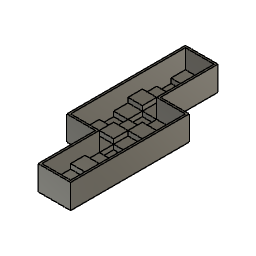
Stepfields v1 (Autodesk Fusion 360 design; units mm, degrees)
Autodesk Fusion 360 part; units mm, degrees
sketch "Sketch1" plane through (0, 0, 0) normal (0, 0, 1) x (1, 0, 0)
  line L0 (0, 0) -> (300, 0)
  line L1 (300, 0) -> (300, 1200)
  line L2 (300, 1200) -> (0, 1200)
  line L3 (0, 600) -> (-300, 600)
  line L4 (-300, 600) -> (-300, 1800)
  line L5 (-300, 1800) -> (0, 1800)
  line L6 (0, 1800) -> (0, 1200)
  line L7 (0, 0) -> (0, 600)
  line L8 (20, 1820) -> (20, 1220)
  line L9 (320, 1220) -> (20, 1220)
  line L10 (320, -20) -> (320, 1220)
  line L11 (-20, -20) -> (320, -20)
  line L12 (-20, -20) -> (-20, 580)
  line L13 (-20, 580) -> (-320, 580)
  line L14 (-320, 580) -> (-320, 1820)
  line L15 (-320, 1820) -> (20, 1820)
  dimension "d1" = 300
  dimension "d2" = 1200
  dimension "d3" = 300
  dimension "d4" = 1200
  dimension "d5" = -20
  constraint horizontal L0
  constraint vertical L1
  constraint horizontal L2
  constraint coincident L0.start L7.start
  constraint perpendicular L3 L4
  constraint perpendicular L4 L5
  constraint perpendicular L2 L6
  constraint perpendicular L3 L7
  measures "d1" distance of L0.start L0.end
  measures "d2" distance of L0.end L1.end
  measures "d3" distance of L3.start L3.end
  measures "d4" distance of L3.end L4.end
extrude "Extrude1" add sketch "Sketch1" along normal blind 400 makes body 1
extrude "Extrude2" add sketch "Sketch1" against normal blind 5 separate body contours L0 L1 L2 L3 L4 L5 L6 L7 makes body 2
extrude "Extrude3" add sketch "Sketch1" against normal blind 5 bodies 1 2
extrude "Extrude4" cut 1 faces at (-313.3333, 1400, 400) along direction (0, 0, -1) blind 100 on bodies 1 bodies 1
extrude "Extrude5" cut 1 faces at (-313.3333, 1400, 300) along direction (0, 0, -1) blind 50 on bodies 1 bodies 1
sketch "Sketch2" plane through (0, 0, 0) normal (0, 0, 1) x (1, 0, 0)
  line L0 (0, 0) -> (150, 0)
  line L1 (150, 0) -> (150, 150)
  line L2 (150, 150) -> (0, 150)
  line L3 (0, 150) -> (0, 0)
  line L4 (150, 150) -> (300, 150)
  line L5 (300, 150) -> (300, 0)
  line L6 (300, 0) -> (150, 0)
  line L7 (0, 300) -> (150, 300)
  line L8 (0, 150) -> (0, 300)
  line L9 (150, 300) -> (150, 150)
  line L10 (300, 300) -> (150, 300)
  line L11 (300, 150) -> (300, 300)
  line L12 (150, 600) -> (150, 450)
  line L13 (150, 450) -> (0, 450)
  line L14 (150, 450) -> (300, 450)
  line L15 (150, 300) -> (150, 450)
  line L16 (0, 600) -> (150, 600)
  line L17 (0, 450) -> (0, 600)
  line L18 (300, 600) -> (150, 600)
  line L19 (0, 450) -> (0, 300)
  line L20 (300, 450) -> (300, 300)
  line L21 (300, 450) -> (300, 600)
  line L22 (0, 1200) -> (150, 1200)
  line L23 (0, 1050) -> (0, 900)
  line L24 (300, 1200) -> (150, 1200)
  line L25 (150, 900) -> (150, 1050)
  line L26 (150, 750) -> (0, 750)
  line L27 (0, 900) -> (150, 900)
  line L28 (300, 1050) -> (300, 1200)
  line L29 (150, 900) -> (150, 750)
  line L30 (0, 750) -> (0, 900)
  line L31 (300, 750) -> (300, 600)
  line L32 (150, 1050) -> (0, 1050)
  line L33 (150, 750) -> (300, 750)
  line L34 (300, 1050) -> (300, 900)
  line L35 (150, 1050) -> (300, 1050)
  line L36 (150, 600) -> (150, 750)
  line L37 (0, 1050) -> (0, 1200)
  line L38 (300, 900) -> (150, 900)
  line L39 (300, 750) -> (300, 900)
  line L40 (150, 1200) -> (150, 1050)
  line L41 (0, 750) -> (0, 600)
  line L42 (-150, 900) -> (-150, 750)
  line L43 (0, 900) -> (-150, 900)
  line L44 (-150, 750) -> (0, 750)
  line L45 (-150, 600) -> (-150, 750)
  line L46 (-150, 900) -> (-150, 1050)
  line L47 (-300, 1200) -> (-150, 1200)
  line L48 (-300, 750) -> (-300, 900)
  line L49 (-300, 1050) -> (-300, 1200)
  line L50 (-150, 1050) -> (0, 1050)
  line L51 (-150, 1050) -> (-300, 1050)
  line L52 (-300, 1050) -> (-300, 900)
  line L53 (0, 1200) -> (-150, 1200)
  line L54 (-150, 1200) -> (-150, 1050)
  line L55 (0, 600) -> (-150, 600)
  line L56 (-300, 900) -> (-150, 900)
  line L57 (-300, 750) -> (-300, 600)
  line L58 (-300, 600) -> (-150, 600)
  line L59 (-300, 1650) -> (-300, 1800)
  line L60 (-300, 1650) -> (-300, 1500)
  line L61 (0, 1650) -> (0, 1500)
  line L62 (-150, 1650) -> (0, 1650)
  line L63 (-150, 1500) -> (-150, 1650)
  line L64 (-300, 1350) -> (-300, 1500)
  line L65 (-150, 1500) -> (-150, 1350)
  line L66 (0, 1350) -> (0, 1500)
  line L67 (-150, 1350) -> (-300, 1350)
  line L68 (0, 1350) -> (0, 1200)
  line L69 (-300, 1350) -> (-300, 1200)
  line L70 (-150, 1800) -> (-150, 1650)
  line L71 (-300, 1500) -> (-150, 1500)
  line L72 (0, 1500) -> (-150, 1500)
  line L73 (-150, 1350) -> (0, 1350)
  line L74 (-300, 1800) -> (-150, 1800)
  line L75 (-150, 1200) -> (-150, 1350)
  line L76 (0, 1800) -> (-150, 1800)
  line L77 (0, 1650) -> (0, 1800)
  line L78 (-300, 750) -> (-150, 750)
  line L79 (-300, 1650) -> (-150, 1650)
  point P0 (0, 1200)
  point P1 (150, 600)
  point P2 (0, 900)
  point P3 (0, 600)
  point P4 (0, 750)
  point P5 (-150, 600)
  point P6 (-150, 750)
  point P7 (0, 1050)
  point P8 (0, 1350)
  point P9 (-150, 1200)
  point P10 (0, 1500)
  point P11 (-150, 1800)
  point P12 (-150, 1650)
  point P13 (0, 1200)
  point P14 (0, 1200)
  dimension "d16" = 150
  dimension "d17" = 150
  constraint horizontal L0
  constraint vertical L1
  constraint horizontal L2
  constraint vertical L3
  constraint coincident L0.start L3.end
  constraint symmetric L0.start L1 L5.end
  constraint symmetric L0.end L1 L6.end
  constraint symmetric L2.start L1 L4.start
  constraint symmetric L2.end L1 L4.end
  constraint symmetric L0.start L2 L7.start
  constraint symmetric L0.end L2 L7.end
  constraint symmetric L1.end L2 L4.start
  constraint symmetric L3.start L2 L8.start
  constraint symmetric L2 L4.end L5.start
  constraint symmetric L2 L5.end L10.start
  constraint symmetric L2 L0.end L7.end
  constraint symmetric L0.start L7 P3
  constraint symmetric L0.end L7 P1
  constraint symmetric L1.end L7 L12.end
  constraint symmetric L2.end L7 L13.end
  constraint symmetric L4.end L7 L14.end
  constraint symmetric L5.end L7 L18.start
  constraint symmetric L8.end L7 L19.end
  constraint symmetric L9.start L7 L10.end
  constraint symmetric L7 L2.end L13.end
  constraint symmetric L7 L1.end L12.end
  constraint symmetric L7 L10.start L11.end
  constraint symmetric L7 L4.end L14.end
  constraint symmetric L0.start L16 P14
  constraint symmetric L0.end L16 L22.end
  constraint symmetric L1.end L16 L25.end
  constraint symmetric L2.end L16 P7
  constraint symmetric L4.end L16 L28.start
  constraint symmetric L5.end L16 L24.start
  constraint symmetric L7.start L16 P2
  constraint symmetric L7.end L16 L25.start
  constraint symmetric L10.start L16 L34.end
  constraint symmetric P1 L16 L12.start
  constraint symmetric L12.end L16 L26.start
  constraint symmetric L13.end L16 P4
  constraint symmetric L14.end L16 L31.start
  constraint symmetric P3 L16 L17.end
  constraint symmetric L16 L18.start L21.end
  constraint symmetric L16 P1 L12.start
  constraint symmetric L16 L13.end P4
  constraint symmetric L16 L7.start P2
  constraint symmetric L16 L14.end L31.start
  constraint symmetric L16 L10.start L34.end
  constraint symmetric P1 L30 P5
  constraint symmetric P3 L30 L16.start
  constraint symmetric L18.start L30 L57.end
  constraint symmetric P14 L30 P13
  constraint symmetric P7 L30 L23.start
  constraint symmetric L25.end L30 L46.end
  constraint symmetric L22.end L30 P9
  constraint symmetric L34.end L30 L48.end
  constraint symmetric L25.start L30 L42.start
  constraint symmetric L28.start L30 L49.start
  constraint symmetric P4 L30 L26.end
  constraint symmetric L26.start L30 P6
  constraint symmetric P2 L30 L23.end
  constraint symmetric L31.start L30 L48.start
  constraint symmetric L24.start L30 L47.start
  constraint symmetric P14 L47 P13
  constraint symmetric P7 L47 P8
  constraint symmetric P4 L47 L61.start
  constraint symmetric P2 L47 P10
  constraint symmetric P3 L47 L76.start
  constraint symmetric P5 L47 P11
  constraint symmetric L49.start L47 L64.start
  constraint symmetric L46.end L47 L65.end
  constraint symmetric P6 L47 P12
  constraint symmetric L48.start L47 L59.start
  constraint symmetric P9 L47 L53.end
  constraint symmetric L48.end L47 L60.end
  constraint symmetric L42.start L47 L63.start
  constraint symmetric L49.end L47 L69.end
  constraint symmetric L47 P14 P13
  constraint symmetric L47 L57.end L59.end
  measures "d16" distance of L0.start L0.end
  measures "d17" distance of L0.end L1.end
extrude "Extrude6" add sketch "Sketch2" along normal blind 50 separate body contours L59 L70 L74 L79 makes body 3
extrude "Extrude7" add sketch "Sketch2" along normal blind 50 separate body contours L64 L65 L67 L71 makes body 4
extrude "Extrude8" add sketch "Sketch2" along normal blind 100 contours L47 L67 L69 L75 bodies 4
extrude "Extrude9" add sketch "Sketch2" along normal blind 50 contours L47 L49 L51 L54 bodies 4
extrude "Extrude10" add sketch "Sketch2" along normal blind 50 separate body contours L42 L48 L56 L78 makes body 5
extrude "Extrude11" add sketch "Sketch2" along normal blind 100 contours L45 L57 L58 L78 bodies 5
extrude "Extrude12" add sketch "Sketch2" along normal blind 50 separate body contours L61 L62 L63 L72 makes body 6
extrude "Extrude13" add sketch "Sketch2" along normal blind 100 contours L65 L66 L72 L73 bodies 6 4
extrude "Extrude14" add sketch "Sketch2" along normal blind 50 separate body contours L53 L68 L73 L75 makes body 7
extrude "Extrude15" add sketch "Sketch2" along normal blind 50 separate body contours L23 L43 L46 L50 makes body 8
extrude "Extrude16" add sketch "Sketch2" along normal blind 100 contours L30 L42 L43 L44 bodies 8 5
extrude "Extrude17" add sketch "Sketch2" along normal blind 50 separate body contours L41 L44 L45 L55 makes body 9
extrude "Extrude18" add sketch "Sketch2" along normal blind 50 separate body contours L22 L32 L37 L40 makes body 10
extrude "Extrude19" add sketch "Sketch2" along normal blind 100 contours L24 L28 L35 L40 bodies 10
extrude "Extrude20" add sketch "Sketch2" along normal blind 50 contours L25 L34 L35 L38 bodies 10
extrude "Extrude21" add sketch "Sketch2" along normal blind 50 separate body contours L18 L31 L33 L36 makes body 11
extrude "Extrude22" add sketch "Sketch2" along normal blind 100 contours L12 L14 L18 L21 bodies 11
extrude "Extrude23" add sketch "Sketch2" along normal blind 50 contours L10 L14 L15 L20 bodies 11
extrude "Extrude24" add sketch "Sketch2" along normal blind 50 separate body contours L1 L4 L5 L6 makes body 12
extrude "Extrude25" add sketch "Sketch2" along normal blind 100 separate body contours L23 L25 L27 L32 makes body 13
extrude "Extrude26" add sketch "Sketch2" along normal blind 50 contours L26 L27 L29 L30 bodies 13 8 9 10 11
extrude "Extrude27" add sketch "Sketch2" along normal blind 50 separate body contours L12 L13 L16 L17 makes body 14
extrude "Extrude28" add sketch "Sketch2" along normal blind 100 contours L7 L13 L15 L19 bodies 14 13
extrude "Extrude29" add sketch "Sketch2" along normal blind 50 separate body contours L2 L7 L8 L9 makes body 15
